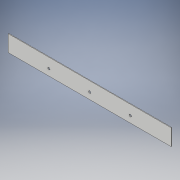
# Autodesk Inventor part: Panel_5x50cm
Saved by Autodesk Inventor 2019 (Build 230136000, 136)
## iProperties
Created: 2018-10-17
Part Number: Panel_5x50cm
Material: Generic
Document SubType Name: Modeling
Designer: nomol
Density: 1 g/cm^3
Appearance: Default
Author: nomol
Autodesk Inventor part; units mm, degrees
ref_plane "YZ Plane" through (0, 0, 0) normal (1, 0, 0) x (0, 1, 0)
ref_plane "XZ Plane" through (0, 0, 0) normal (0, 1, 0) x (-1, 0, 0)
ref_plane "XY Plane" through (0, 0, 0) normal (0, 0, 1) x (1, 0, 0)
sketch "Sketch3" plane through (0, 0, 0) normal (0, 0, 1) x (1, 0, 0)
  line L0 (0, 0) -> (500, 0)
  line L1 (500, 0) -> (500, 50)
  line L2 (500, 50) -> (0, 50)
  line L3 (0, 50) -> (0, 0)
  dimension "d5" = 50
  dimension "d6" = 500
  constraints: 8 end point, 2 parallel, 1 horizontal, 1 perpendicular
  measures "d5" distance of L0.end L1.end
  measures "d6" distance of L1.end L2.end
extrude "Extrusion3" add sketch "Sketch3" along normal blind 2
sketch "Sketch6" plane through (0, 0, 2) normal (0, 0, 1) x (1, 0, 0)
  circle A0 centre (125, 20) radius 3.57
  line L0 (0, 0) -> (500, 0) projected
  circle A1 centre (250, 20) radius 3.57
  circle A2 centre (375, 20) radius 3.57
  line L1 (0, 50) -> (0, 0) projected
  line L2 (500, 0) -> (500, 50) projected
  dimension "d19" = 7.14
  dimension "d22" = 20
  dimension "d23" = 7.14
  dimension "d24" = 7.14
  dimension "d25" = 125
  dimension "d26" = 20
  dimension "d27" = 250
  dimension "d28" = 20
  dimension "d29" = 125
  constraints: 3 centre point
  measures "d19" diameter of A0
  measures "d22" distance from line of L0 A0.centre
  measures "d23" diameter of A1
  measures "d24" diameter of A2
  measures "d25" distance from line of L1 A0.centre
  measures "d26" distance from line of L0 A1.centre
  measures "d27" distance from line of L2 A1.centre
  measures "d28" distance from line of L0 A2.centre
  measures "d29" distance from line of L2 A2.centre
extrude "Extrusion4" cut sketch "Sketch6" against normal up to next
body "Solid3"
